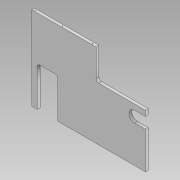
# Autodesk Inventor part: Bottom
Saved by Autodesk Inventor 2021.4 (Build 254397000, 397)
## iProperties
Created: 2022-05-18
Part Number: Bottom
Material: Generic
Document SubType Name: Modeling
Designer: LaborAdmin
Density: 1 g/cm^3
Appearance: Default
Author: LaborAdmin
Autodesk Inventor part; units mm, degrees
ref_plane "YZ Plane" through (0, 0, 0) normal (1, 0, 0) x (0, 1, 0)
ref_plane "XZ Plane" through (0, 0, 0) normal (0, 1, 0) x (-1, 0, 0)
ref_plane "XY Plane" through (0, 0, 0) normal (0, 0, 1) x (1, 0, 0)
sketch "Sketch1" plane through (0, 0, 0) normal (0, 0, 1) x (1, 0, 0)
  line L0 (-207.5, -152.5) -> (207.5, -152.5)
  line L1 (207.5, -152.5) -> (207.5, 152.5)
  line L2 (207.5, 152.5) -> (-207.5, 152.5)
  line L3 (-207.5, 152.5) -> (-207.5, -152.5)
  line L4 (-207.5, -152.5) -> (207.5, 152.5) construction
  line L5 (207.5, -152.5) -> (-207.5, 152.5) construction
  point P0 (0, 0)
  dimension "d0" = 415
  dimension "d1" = 305
  constraints: 12 end point, 2 midpoint, 2 parallel, 1 horizontal, 1 perpendicular
  measures "d0" distance of L1.end L2.end
  measures "d1" distance of L2.end L0.start
extrude "Extrusion1" add sketch "Sketch1" along normal blind 10
sketch "Sketch2" plane through (0, 0, 10) normal (0, 0, 1) x (1, 0, 0)
  line L0 (-207.5, -152.5) -> (207.5, -152.5) projected
  line L1 (-187.5, -152.5) -> (-112.5, -152.5)
  line L2 (-112.5, -152.5) -> (-112.5, -17.5)
  line L3 (-122.5, -7.5) -> (-177.5, -7.5)
  line L4 (-187.5, -17.5) -> (-187.5, -152.5)
  line L5 (-207.5, 152.5) -> (-207.5, -152.5) projected
  line L6 (207.5, -152.5) -> (207.5, 152.5) projected
  line L7 (207.5, 22.5) -> (167.5, 22.5)
  line L8 (167.5, 22.5) -> (167.5, -17.5) construction
  line L9 (167.5, -17.5) -> (207.5, -17.5)
  line L10 (207.5, -17.5) -> (207.5, 22.5)
  line L11 (207.5, 152.5) -> (-207.5, 152.5) projected
  arc A0 (167.5, 22.5) -> (167.5, -17.5) centre (167.5, 2.5) ccw
  line L12 (27.5, 152.5) -> (207.5, 152.5)
  line L13 (207.5, 152.5) -> (207.5, 42.5)
  line L14 (207.5, 42.5) -> (37.5, 42.5)
  line L15 (27.5, 52.5) -> (27.5, 152.5)
  arc A1 (-177.5, -7.5) -> (-187.5, -17.5) centre (-177.5, -17.5) ccw
  arc A2 (-112.5, -17.5) -> (-122.5, -7.5) centre (-122.5, -17.5) ccw
  arc A3 (27.5, 52.5) -> (37.5, 42.5) centre (37.5, 52.5) ccw
  point P0 (0, 0)
  point P1 (-112.5, -7.5)
  point P2 (-187.5, -7.5)
  point P3 (27.5, 42.5)
  dimension "d4" = 145
  dimension "d5" = 75
  dimension "d6" = 20
  dimension "d7" = 40
  dimension "d8" = 40
  dimension "d9" = 130
  dimension "d10" = 110
  dimension "d11" = 180
  dimension "d41" = 10
  constraints: 24 end point, 10 point on line, 8 point on circle, 7 tangent, 6 parallel, 4 centre point, 3 horizontal, 3 perpendicular, 2 equal radius, 1 midpoint
  measures "d4" distance of point (-187.5, -7.5) L1.start
  measures "d5" distance of point (-112.5, -7.5) point (-187.5, -7.5)
  measures "d6" distance between parallel lines of L5 L4
  measures "d7" distance of L7.end L8.end
  measures "d8" distance of L7.start L7.end
  measures "d9" distance between parallel lines of L11 L7
  measures "d10" distance of point (27.5, 42.5) L12.start
  measures "d11" distance of L13.end point (27.5, 42.5)
  measures "d41" radius of A1
extrude "Extrusion2" cut sketch "Sketch2" against normal blind 10 contours L4 A1 L3 A2 L2 L0 | L11 L6 L14 A3 L15 | L9 A0 L7 L6
sketch "Sketch3" plane through (207.5, -152.5, 0) normal (0, -1, 0) x (1, 0, 0)
  line L0 (-415, 0) -> (-415, 10) projected
  line L1 (-415, 6) -> (0, 6) construction
  line L2 (0, 10) -> (0, 0) projected
  line L3 (-320, 0) -> (0, 0) construction
  line L4 (-395, 0) -> (-395, 10) construction
  point P0 (-207.5, 0)
  point P1 (-407, 6)
  point P2 (-307, 6)
  point P3 (-37, 6)
  point P4 (-157, 6)
  dimension "d14" = 6
  dimension "d15" = 415
  dimension "d16" = 20
  dimension "d17" = 8
  dimension "d18" = 100
  dimension "d19" = 150
  dimension "d20" = 120
  constraints: 6 point on line, 2 end point, 1 horizontal
  measures "d14" distance between parallel lines of L3 L1
  measures "d15" distance between parallel lines of L2 L0
  measures "d16" distance between parallel lines of L4 L0
  measures "d17" distance from line of L0 point (-407, 6)
  measures "d18" distance of point (-307, 6) point (-407, 6)
  measures "d19" distance of point (-157, 6) point (-307, 6)
  measures "d20" distance of point (-37, 6) point (-157, 6)
sketch "Sketch4" plane through (-207.5, 152.5, 10) normal (0, 1, 0) x (1, 0, 0)
  line L0 (0, 10) -> (0, 0) projected
  line L1 (0, 4) -> (235, 4) construction
  line L2 (235, 10) -> (0, 10) projected
  point P0 (207.5, 10)
  point P1 (8, 4)
  point P2 (108, 4)
  point P3 (218, 4)
  dimension "d22" = 6
  dimension "d23" = 8
  dimension "d24" = 210
  dimension "d25" = 100
  constraints: 4 point on line, 2 end point, 1 horizontal, 1 vertical alignment
  measures "d22" distance between parallel lines of L1 L2
  measures "d23" distance of L1.start point (8, 4)
  measures "d24" distance of point (218, 4) point (8, 4)
  measures "d25" distance of point (8, 4) point (108, 4)
hole "Hole1" at (-199.5, -152.5, 6) at (-99.5, -152.5, 6) at (50.5, -152.5, 6) at (170.5, -152.5, 6) direction (0, 1, 0) diameter 2.459 depth 10 thread size "M3x0.5" designation "M3" class "6H" standard "ISO Metric profile"
hole "Hole2" at (10.5, 152.5, 6) at (-99.5, 152.5, 6) at (-199.5, 152.5, 6) direction (0, -1, 0) diameter 2.459 depth 10 thread size "M3x0.5" designation "M3" class "6H" standard "ISO Metric profile"
body "Solid1"
